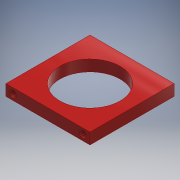
# Autodesk Inventor part: SpacerSmall
Saved by Autodesk Inventor 2019.3 (Build 233278000, 278)
## iProperties
Created: 2018-09-29
Part Number: SpacerSmall
Material: Generic
Document SubType Name: Modeling
Designer: eroldan
Density: 1 g/cm^3
Appearance: Default
Author: eroldan
Autodesk Inventor part; units mm, degrees
ref_plane "YZ Plane" through (0, 0, 0) normal (1, 0, 0) x (0, 1, 0)
ref_plane "XZ Plane" through (0, 0, 0) normal (0, 1, 0) x (-1, 0, 0)
ref_plane "XY Plane" through (0, 0, 0) normal (0, 0, 1) x (1, 0, 0)
sketch "Sketch1" plane through (0, 0, 0) normal (0, 0, 1) x (1, 0, 0)
  line L0 (-30, -30) -> (30, -30)
  line L1 (30, -30) -> (30, 30)
  line L2 (30, 30) -> (-30, 30)
  line L3 (-30, 30) -> (-30, -30)
  line L4 (-30, -30) -> (30, 30) construction
  line L5 (30, -30) -> (-30, 30) construction
  point P0 (0, 0)
  dimension "d0" = 60
  dimension "d1" = 60
  constraints: 12 end point, 2 midpoint, 2 parallel, 1 horizontal, 1 perpendicular
  measures "d0" distance of L2.end L1.end
  measures "d1" distance of L1.end L0.end
extrude "Extrusion1" add sketch "Sketch1" along normal blind 8
hole "Hole1" at (0, 0, 0) direction (0, 0, 1) diameter 43 end through all
sketch "Sketch2" plane through (-30, 30, 0) normal (0, 1, 0) x (1, 0, 0)
  line L0 (60, 0) -> (0, 0) projected
  line L1 (0, 0) -> (0, -8) projected
  line L2 (60, -8) -> (0, -8) projected
  line L3 (60, 0) -> (60, -8) projected
  point P0 (30, 0)
  point P1 (55, -4)
  point P2 (5, -4)
  dimension "d11" = 5
  dimension "d12" = 5
  measures "d11" distance from line of L3 point (55, -4)
  measures "d12" distance from line of L1 point (5, -4)
hole "Hole2" at (-25, 30, 4) at (25, 30, 4) direction (0, -1, 0) diameter 5 end through all
equation "\"d12\" = d11"
body "Solid1"
